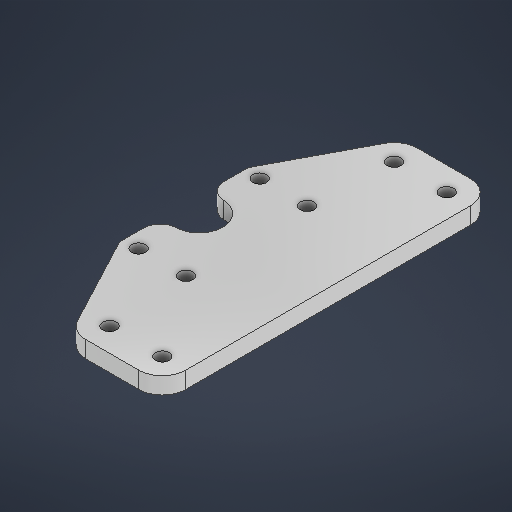
# Autodesk Inventor part: CNC-001-StructureGusset2
Saved by Autodesk Inventor 2026.2 (Build 302298000, 298)
## iProperties
Created: 2026-06-14
Part Number: CNC-001-StructureGusset2
Material: Aluminum 6061
Document SubType Name: Modeling
Designer: Kenji
Density: 2.7 g/cm^3
Appearance: Aluminum - Dark
Author: Kenji
Autodesk Inventor part; units mm, degrees
ref_plane "YZ Plane" through (0, 0, 0) normal (1, 0, 0) x (0, 1, 0)
ref_plane "XZ Plane" through (0, 0, 0) normal (0, 1, 0) x (-1, 0, 0)
ref_plane "XY Plane" through (0, 0, 0) normal (0, 0, 1) x (1, 0, 0)
sketch "Sketch1" plane through (0, 0, 0) normal (0, 1, 0) x (-1, 0, 0)
  circle A0 centre (0, 0) radius 2.6
  line L0 (0, 0) -> (2.6, 0) construction
  circle A1 centre (20, 0) radius 2.6
  circle A2 centre (22, -31) radius 2.6
  line L1 (22, -31) -> (24.6, -31) construction
  line L2 (22, -31) -> (22, -33.6) construction
  circle A3 centre (40, -31) radius 2.6
  circle A4 centre (22, -77) radius 2.6
  circle A5 centre (40, -77) radius 2.6
  circle A6 centre (20, -108) radius 2.6
  circle A7 centre (0, -108) radius 2.6
  circle A8 centre (20, 0) radius 8.95 construction
  circle A9 centre (0, 0) radius 8.95 construction
  circle A10 centre (20, -108) radius 8.95 construction
  circle A11 centre (0, -108) radius 8.95 construction
  circle A12 centre (40, -31) radius 5.775 construction
  circle A13 centre (40, -77) radius 5.775 construction
  line L3 (27.9103, 4.1868) -> (45.1042, -28.2985)
  line L4 (45.1042, -79.7015) -> (27.9103, -112.1868)
  line L5 (-8.95, 0) -> (-8.95, -108)
  line L6 (20, 8.95) -> (0, 8.95)
  line L7 (20, -116.95) -> (0, -116.95)
  line L8 (45.775, -31) -> (45.775, -77)
  arc A14 (45.1042, -79.7015) -> (45.775, -77) centre (40, -77) ccw
  arc A15 (45.775, -31) -> (45.1042, -28.2985) centre (40, -31) ccw
  arc A16 (27.9103, 4.1868) -> (20, 8.95) centre (20, 0) ccw
  arc A17 (0, 8.95) -> (-8.95, 0) centre (0, 0) ccw
  arc A18 (-8.95, -108) -> (0, -116.95) centre (0, -108) ccw
  arc A19 (20, -116.95) -> (27.9103, -112.1868) centre (20, -108) ccw
  point P0 (42.6, -31)
  point P1 (40, -33.6)
  point P2 (24.6, -77)
  point P3 (22, -79.6)
  point P4 (42.6, -77)
  point P5 (40, -79.6)
  dimension "d0" = 5.2
  dimension "d1" = 20
  dimension "d2" = 31
  dimension "d3" = 22
  dimension "d6" = 18
  dimension "d9" = 46
  dimension "d12" = 31
  dimension "d13" = 6.35
  dimension "d14" = 3.175
  constraints: 33 point on circle, 19 centre point, 18 end point, 11 tangent, 6 coincident, 6 equal radius, 5 concentric, 5 horizontal, 2 horizontal alignment, 2 point on line, 2 vertical, 2 vertical alignment, 1 perpendicular, 16 other
  measures "d1" distance of point (0, 0) A1.centre
  measures "d2" vertical distance of L1.start point (0, 0)
  measures "d3" horizontal distance of point (0, 0) L1.start
  measures "d6" distance of L1.start A3.centre
  measures "d9" distance of L1.start A4.centre
  measures "d12" vertical distance of A6.centre A4.centre
  measures "d13" radial gap between concentric circles of A1 A8
  measures "d14" radial gap between concentric circles of A12 A3
extrude "Extrusion1" add sketch "Sketch1" along normal blind 6.35
sketch "Sketch2" plane through (0, 6.35, 0) normal (0, 1, 0) x (1, 0, 0)
  arc A0 (0, -8.95) -> (8.95, 0) centre (0, 0) ccw projected
  line L0 (8.95, 0) -> (8.95, 108) projected
  arc A1 (8.95, 108) -> (0, 116.95) centre (0, 108) ccw projected
  line L1 (0, 116.95) -> (-20, 116.95) projected
  arc A2 (-20, 116.95) -> (-27.9103, 112.1868) centre (-20, 108) ccw projected
  line L2 (-27.9103, 112.1868) -> (-45.1042, 79.7015) projected
  arc A3 (-45.1042, 79.7015) -> (-45.775, 77) centre (-40, 77) ccw projected
  line L3 (-45.775, 77) -> (-45.775, 31) projected
  arc A4 (-45.775, 31) -> (-45.1042, 28.2985) centre (-40, 31) ccw projected
  line L4 (-45.1042, 28.2985) -> (-27.9103, -4.1868) projected
  arc A5 (-27.9103, -4.1868) -> (-20, -8.95) centre (-20, 0) ccw projected
  line L5 (-20, -8.95) -> (0, -8.95) projected
  circle A6 centre (-20, 0) radius 2.6 projected
  circle A7 centre (-22, 31) radius 2.6 projected
  circle A8 centre (-40, 31) radius 2.6 projected
  circle A9 centre (-22, 77) radius 2.6 projected
  circle A10 centre (-40, 77) radius 2.6 projected
  circle A11 centre (-20, 108) radius 2.6 projected
  circle A12 centre (0, 108) radius 2.6 projected
  circle A13 centre (0, 0) radius 2.6 projected
  circle A14 centre (-40, 54) radius 9
  point P0 (-45.775, 60.9029)
  point P1 (-45.775, 47.0971)
  dimension "d17" = 18
  dimension "d18" = 46
  dimension "d19" = 23
  constraints: 1 centre point, 1 vertical alignment
  measures "d17" diameter of A14
  measures "d18" distance of A4.centre A10.centre
  measures "d19" distance of A14.centre A3.centre
extrude "Extrusion2" cut sketch "Sketch2" against normal through all contours L3 A14 picked at (-38.3999, 55.6279)
fillet "Fillet1" radius 6.35 2 edges at (-45.775, 3.175, -60.9029) (-45.775, 3.175, -47.0971)
equation "\"d12\" = d2"
equation "\"d19\" = 0.5 * d18"
body "Solid1"
